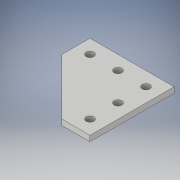
# Autodesk Inventor part: 2020-90-plate
Saved by Autodesk Inventor 2019 (Build 230136000, 136)
## iProperties
Created: 2019-04-21
Part Number: 2020-90-plate
Material: Generic
Document SubType Name: Modeling
Designer: Alex Jones
Density: 1 g/cm^3
Appearance: Default
Author: Alex Jones
Autodesk Inventor part; units mm, degrees
ref_plane "YZ Plane" through (0, 0, 0) normal (1, 0, 0) x (0, 1, 0)
ref_plane "XZ Plane" through (0, 0, 0) normal (0, 1, 0) x (-1, 0, 0)
ref_plane "XY Plane" through (0, 0, 0) normal (0, 0, 1) x (1, 0, 0)
sketch "Sketch1" plane through (0, 0, 0) normal (0, 1, 0) x (-1, 0, 0)
  line L0 (-30, 30) -> (-10, 30)
  line L1 (30, -10) -> (30, -30)
  line L2 (30, -30) -> (-30, -30)
  line L3 (-30, -30) -> (-30, 30)
  line L4 (-30, 30) -> (30, -30) construction
  line L5 (30, 30) -> (-30, -30) construction
  line L6 (-30, 30) -> (-10, 30)
  line L7 (-10, -30) -> (-30, -30)
  line L8 (-30, -30) -> (-30, 30)
  line L9 (30, -30) -> (-10, -30)
  line L10 (30, -10) -> (30, -30)
  line L11 (-10, 30) -> (30, -10)
  circle A0 centre (-20, -20) radius 2.75
  circle A1 centre (-20, 0) radius 2.75
  circle A2 centre (-20, 20) radius 2.75
  circle A3 centre (0, -20) radius 2.75
  circle A4 centre (20, -20) radius 2.75
  point P0 (0, 0)
  dimension "d0" = 60
  dimension "d1" = 60
  dimension "d4" = 5.5
  dimension "d5" = 5.5
  dimension "d6" = 5.5
  dimension "d7" = 5.5
  dimension "d8" = 5.5
  constraints: 24 end point, 5 centre point, 4 parallel, 4 point on line, 3 horizontal, 2 midpoint, 1 perpendicular
  measures "d0" distance of L5.start L1.end
  measures "d1" distance of L1.end L2.end
  measures "d4" diameter of A0
  measures "d5" diameter of A1
  measures "d6" diameter of A2
  measures "d7" diameter of A3
  measures "d8" diameter of A4
extrude "Extrusion1" add sketch "Sketch1" along normal blind 4
body "Solid1"
